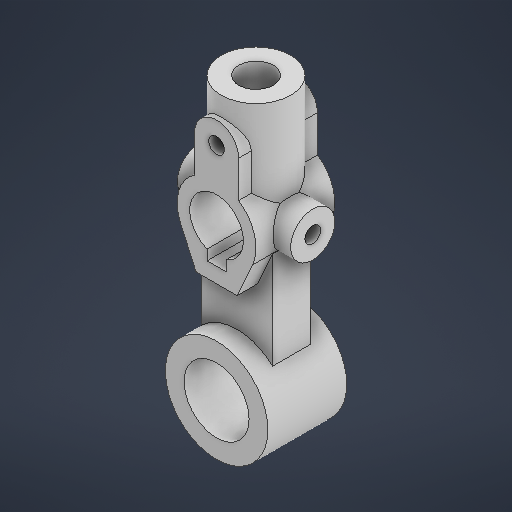
# Autodesk Inventor part: b3
Saved by Autodesk Inventor 2025.4 (Build 294407000, 407)
## iProperties
Created: 2026-05-15
Part Number: b3
Material: Generic
Document SubType Name: Modeling
Designer: VuQuan
Density: 1 g/cm^3
Appearance: Default
Author: VuQuan
Autodesk Inventor part; units mm, degrees
ref_plane "YZ Plane" through (0, 0, 0) normal (1, 0, 0) x (0, 1, 0)
ref_plane "XY Plane" through (0, 0, 0) normal (0, 0, 1) x (1, 0, 0)
sketch "Sketch1" plane through (0, 0, 0) normal (0, 0, 1) x (1, 0, 0)
  circle A0 centre (0, 0) radius 32.5
  circle A1 centre (0, 0) radius 20.625
  line L0 (22.5, 23.4521) -> (22.5, 85.0796)
  line L1 (-22.5, 23.4521) -> (-22.5, 85.0796)
  arc A2 (6, 80.094) -> (-6, 80.094) centre (0, 96) ccw
  line L2 (-22.7923, 85.7281) -> (-13, 64)
  line L3 (-13, 64) -> (13, 64)
  line L4 (13, 64) -> (22.7923, 85.7281)
  line L5 (-6, 80.094) -> (-6, 73.6)
  line L6 (-6, 73.6) -> (6, 73.6)
  line L7 (6, 73.6) -> (6, 80.094)
  line L8 (-14, 116.7123) -> (-14, 140)
  arc A3 (14, 140) -> (-14, 140) centre (0, 140) ccw
  line L9 (14, 140) -> (14, 116.7123)
  circle A4 centre (0, 140) radius 5
  arc A5 (22.7923, 85.7281) -> (14, 116.7123) centre (0, 96) ccw
  arc A6 (-14, 116.7123) -> (-22.7923, 85.7281) centre (0, 96) ccw
  point P0 (0, 64)
  point P1 (0, 73.6)
  dimension "d0" = 65
  dimension "d1" = 41.25
  dimension "d4" = 34
  dimension "d6" = 45
  dimension "d7" = 12
  dimension "d8" = 22.4
  dimension "d9" = 96
  dimension "d10" = 26
  dimension "d11" = 32
  dimension "d12" = 14
  dimension "d13" = 10
  dimension "d14" = 44
  dimension "d15" = 25
  constraints: 20 end point, 10 point on circle, 7 centre point, 4 coincident, 4 tangent, 4 vertical, 4 vertical alignment, 3 parallel, 2 midpoint, 2 perpendicular, 2 point on line, 1 horizontal
  measures "d0" diameter of A0
  measures "d1" diameter of A1
  measures "d4" diameter of A2
  measures "d6" distance between parallel lines of L0 L1
  measures "d7" distance of L5.end L6.end
  measures "d8" distance from line of A2.centre L6
  measures "d9" distance of A2.centre point (0, 0)
  measures "d10" distance of L2.end L3.end
  measures "d11" distance from line of L3 A2.centre
  measures "d12" radius of A3
  measures "d13" diameter of A4
  measures "d14" distance of A2.centre A3.centre
  measures "d15" radius of A5
extrude "Extrusion1" add sketch "Sketch1" along normal mid plane 50 contours A0
extrude "Extrusion2" add sketch "Sketch1" along normal mid plane 24 contours A0 L1 L2 L3 L4 L0
extrude "Extrusion3" add sketch "Sketch1" along normal mid plane 50 contours L4 L3 L2 A6 L8 A3 L9 A5
sketch "Sketch3" plane through (0, 0, 0) normal (1, 0, 0) x (0, 1, 0)
  line L0 (80.094, 25) -> (113, 25) projected
  circle A0 centre (96.547, 0) radius 5
  circle A1 centre (96.547, 0) radius 14
  point P0 (0, 0)
  point P1 (96.547, 25)
  dimension "d20" = 10
  dimension "d21" = 28
  constraints: 2 centre point, 1 coincident, 1 horizontal alignment, 1 midpoint, 1 vertical alignment
  measures "d20" diameter of A0
  measures "d21" diameter of A1
extrude "Extrusion4" add sketch "Sketch3" along normal mid plane 72 contours A0 | A1
extrude "Extrusion5" cut sketch "Sketch1" along normal mid plane 50 contours L7 L6 L5 A2
extrude "Extrusion6" cut sketch "Sketch3" along normal mid plane 72 contours A0
ref_plane "Work Plane1" through (0, 166, 0) normal (0, 1, 0) x (-1, 0, 0)
sketch "Sketch4" plane through (0, 166, 0) normal (0, 1, 0) x (-1, 0, 0)
  circle A0 centre (0, 0) radius 11
  circle A1 centre (0, 0) radius 22
  dimension "d29" = 22
  dimension "d30" = 44
  constraints: 2 centre point, 2 coincident
  measures "d29" diameter of A0
  measures "d30" diameter of A1
extrude "Extrusion7" add sketch "Sketch4" against normal up to next contours A0 | A1
extrude "Extrusion8" cut sketch "Sketch4" against normal up to next contours A0
body "Solid1"
